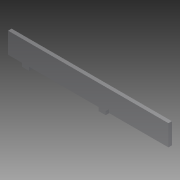
# Autodesk Inventor part: Funneling 3
Saved by Autodesk Inventor 2013 (Build 170138000, 138)
## iProperties
Created: 2013-01-26
Part Number: Funneling 3
Material: Polycarbonate, Clear
Document SubType Name: Modeling
Designer: actoennies
Mass: 64.0939 g
Surface Area: 269.354 cm^2
Volume: 71.6934 cm^3
Density: 0.894 g/cm^3
Author: actoennies
Autodesk Inventor part; units mm, degrees
ref_plane "YZ Plane" through (0, 0, 0) normal (1, 0, 0) x (0, 1, 0)
ref_plane "XZ Plane" through (0, 0, 0) normal (0, 1, 0) x (-1, 0, 0)
ref_plane "XY Plane" through (0, 0, 0) normal (0, 0, 1) x (1, 0, 0)
sketch "Sketch1" plane through (0, 0, 0) normal (0, 0, 1) x (1, 0, 0)
  line L0 (0, 0) -> (0, 38.1)
  line L1 (0, 38.1) -> (292.1, 38.1)
  line L2 (292.1, 38.1) -> (292.1, 0)
  line L3 (0, 0) -> (25.4, 0)
  line L4 (25.4, 0) -> (25.4, -6.35)
  line L5 (25.4, -6.35) -> (38.1, -6.35)
  line L6 (38.1, -6.35) -> (38.1, 0)
  line L7 (38.1, 0) -> (165.1, 0)
  line L8 (165.1, 0) -> (165.1, -6.35)
  line L9 (165.1, -6.35) -> (177.8, -6.35)
  line L10 (177.8, -6.35) -> (177.8, 0)
  line L11 (177.8, 0) -> (292.1, 0)
  dimension "d0" = 38.1
  dimension "d1" = 25.4
  dimension "d3" = 6.35
  dimension "d4" = 12.7
  dimension "d5" = 127
  dimension "d6" = 12.7
  dimension "d7" = 292.1
  constraints: 24 end point, 6 perpendicular, 4 parallel, 1 collinear, 1 vertical
  measures "d0" distance of L0.start L0.end
  measures "d1" distance of L0.start L3.end
  measures "d3" distance of L3.end L4.end
  measures "d4" distance of L4.end L5.end
  measures "d5" distance of L6.end L7.end
  measures "d6" distance of L8.end L9.end
  measures "d7" distance of L0.end L1.end
extrude "Extrusion1" add sketch "Sketch1" along normal blind 6.35
body "Solid1"
